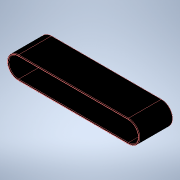
# Autodesk Inventor part: pastran
Saved by Autodesk Inventor 2022 (Build 260153000, 153)
## iProperties
Created: 2023-05-02
Part Number: pastran
Material: Ogólny
Document SubType Name: Modeling
Designer: nosal
Density: 1 g/cm^3
Appearance: Domyślna
Author: nosal
Autodesk Inventor part; units mm, degrees
ref_plane "YZ Plane" through (0, 0, 0) normal (1, 0, 0) x (0, 1, 0)
ref_plane "XZ Plane" through (0, 0, 0) normal (0, 1, 0) x (-1, 0, 0)
ref_plane "XY Plane" through (0, 0, 0) normal (0, 0, 1) x (1, 0, 0)
sketch "Szkic1" plane through (0, 0, 0) normal (0, 0, 1) x (1, 0, 0)
  arc A0 (0, 35) -> (0, -35) centre (0, 0) ccw
  line L0 (0, 35) -> (390, 35)
  arc A1 (390, -35) -> (390, 35) centre (390, 0) ccw
  line L1 (0, -35) -> (390, -35)
  line L2 (390, 40) -> (0, 40)
  arc A2 (0, 40) -> (0, -40) centre (0, 0) ccw
  line L3 (0, -40) -> (390, -40)
  arc A3 (390, -40) -> (390, 40) centre (390, 0) ccw
  point P0 (424.991, -0.7958)
  dimension "d0" = 70
  dimension "d1" = 390
  dimension "d2" = 70
  dimension "d3" = 5
  constraints: 9 point on circle, 8 end point, 4 centre point, 2 horizontal, 2 tangent, 1 coincident, 3 other
  measures "d0" diameter of A0
  measures "d1" distance of L0.start L0.end
  measures "d2" diameter of A1
  measures "d3" distance between parallel lines of L2 L0
extrude "Wyciągnięcie proste1" add sketch "Szkic1" along normal blind 120
fillet "Zaokrąglenie1" radius 2 4 edges at (-40, 0, 120) (195, -40, 120) (430, 0, 120) (195, 40, 120)
fillet "Zaokrąglenie2" radius 2 4 edges at (195, 35, 120) (425, 0, 120) (195, -35, 120) (-35, 0, 120)
fillet "Zaokrąglenie3" radius 2 4 edges at (-40, 0, 0) (195, -40, 0) (430, 0, 0) (195, 40, 0)
fillet "Zaokrąglenie4" radius 2 4 edges at (425, 0, 0) (195, -35, 0) (-35, 0, 0) (195, 35, 0)
